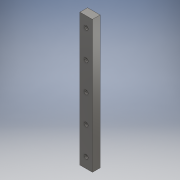
# Autodesk Inventor part: slider_b5p5x9_95_sa
Saved by Autodesk Inventor 2018 (Build 220112000, 112)
## iProperties
Created: 2018-02-23
Part Number: slider_b5p5x9_95_sa
Material: ステンレス鋼
Document SubType Name: Modeling
Designer: shun
Density: 8 g/cm^3
Appearance: 半つや出し
Author: shun
Autodesk Inventor part; units mm, degrees
ref_plane "YZ Plane" through (0, 0, 0) normal (1, 0, 0) x (0, 1, 0)
ref_plane "XZ Plane" through (0, 0, 0) normal (0, 1, 0) x (-1, 0, 0)
ref_plane "XY Plane" through (0, 0, 0) normal (0, 0, 1) x (1, 0, 0)
sketch "スケッチ1" plane through (0, 0, 0) normal (0, 0, 1) x (1, 0, 0)
  line L0 (4.5, -2.75) -> (-4.5, -2.75)
  line L1 (-4.5, -2.75) -> (-4.5, 2.75)
  line L2 (-4.5, 2.75) -> (4.5, 2.75)
  line L3 (4.5, 2.75) -> (4.5, -2.75)
  line L4 (4.5, -2.75) -> (-4.5, 2.75) construction
  line L5 (-4.5, -2.75) -> (4.5, 2.75) construction
  point P0 (0, 0)
  dimension "d0" = 9
  dimension "d1" = 5.5
  constraints: 12 end point, 2 midpoint, 2 parallel, 1 horizontal, 1 perpendicular
  measures "d0" distance of L1.end L2.end
  measures "d1" distance of L0.end L1.end
extrude "押し出し1" add sketch "スケッチ1" along normal blind 95
sketch "スケッチ2" plane through (-4.5, 2.75, 0) normal (0, 1, 0) x (1, 0, 0)
  point P0 (4.5, 0)
  point P1 (4.5, -7.5)
  point P2 (4.5, -27.5)
  point P3 (4.5, -47.5)
  point P4 (4.5, -67.5)
  point P5 (4.5, -87.5)
  dimension "d4" = 47.5
  dimension "d5" = 20
  dimension "d6" = 20
  dimension "d7" = 20
  dimension "d8" = 20
  measures "d4" distance of point (4.5, 0) point (4.5, -47.5)
  measures "d5" distance of point (4.5, -27.5) point (4.5, -47.5)
  measures "d6" distance of point (4.5, -7.5) point (4.5, -27.5)
  measures "d7" distance of point (4.5, -67.5) point (4.5, -47.5)
  measures "d8" distance of point (4.5, -67.5) point (4.5, -87.5)
hole "穴1" at (0, 2.75, 7.5) at (0, 2.75, 27.5) at (0, 2.75, 47.5) at (0, 2.75, 67.5) at (0, 2.75, 87.5) direction (0, -1, 0) diameter 3 end through all
equation "\"d6\" = d5"
equation "\"d7\" = d5"
equation "\"d8\" = d5"
